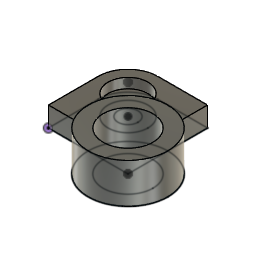
6주_예제#3 (Autodesk Fusion 360 design; units mm, degrees)
Autodesk Fusion 360 part; units mm, degrees
note: some values were not read from the file. Set by a fixed rule: which sketch regions a step uses.
sketch "스케치1" plane through (0, 0, 0) normal (0, 0, 1) x (1, 0, 0)
  line L0 (0, 0) -> (40, 0)
  line L1 (40, 0) -> (40, 40)
  line L2 (40, 40) -> (15, 40)
  line L3 (0, 25) -> (0, 0)
  circle A0 centre (40, 0) radius 20
  circle A1 centre (40, 0) radius 12.5
  arc A2 (15, 40) -> (0, 25) centre (15, 25) ccw
  circle A3 centre (15, 25) radius 10
  circle A4 centre (15, 25) radius 5
  point P0 (0, 40)
  dimension "d1" = 40
  dimension "d2" = 40
  dimension "d3" = 40
  dimension "d4" = 25
  dimension "d5" = 15
  dimension "d6" = 20
  dimension "d7" = 10
  constraint horizontal L0
  constraint vertical L1
  constraint horizontal L2
  constraint vertical L3
  constraint coincident L0.start L3.end
  constraint coincident L0.end L1.start
  constraint concentric A0 A1
  constraint coincident P0 L2
  constraint coincident P0 L3
  constraint tangent L2 A2
  constraint tangent L3 A2
  constraint concentric A2 A3
  constraint concentric A2 A4
  measures "d1" distance of L0.start L0.end
  measures "d2" distance of L0.start P0
  measures "d3" diameter of A0
  measures "d4" diameter of A1
  measures "d5" radius of A2
  measures "d6" diameter of A3
  measures "d7" diameter of A4
extrude "돌출4" add sketch "스케치1" along normal blind 5 contours A3
extrude "돌출5" add sketch "스케치1" along normal blind 10 contours L0 L1 L2 L3 A0 A2
extrude "돌출6" add sketch "스케치1" along normal blind 20 contours L0 L1 A0 A1 | L0 L1 A0 A1
